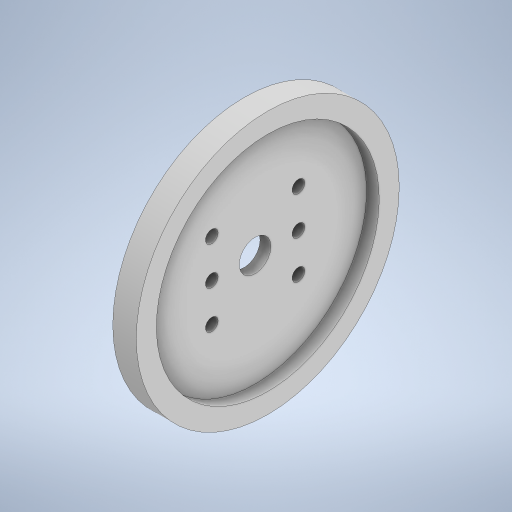
# Autodesk Inventor part: 4ax_plate_joint
Saved by Autodesk Inventor 2024 (Build 280153000, 153)
## iProperties
Created: 2025-12-19
Part Number: 4ax_plate_joint
Material: Generic
Document SubType Name: Modeling
Designer: schar
Density: 1 g/cm^3
Appearance: Default
Author: schar
Autodesk Inventor part; units mm, degrees
ref_plane "YZ Plane" through (0, 0, 0) normal (1, 0, 0) x (0, 1, 0)
ref_plane "XZ Plane" through (0, 0, 0) normal (0, 1, 0) x (-1, 0, 0)
ref_plane "XY Plane" through (0, 0, 0) normal (0, 0, 1) x (1, 0, 0)
sketch "Sketch1" plane through (0, 0, 0) normal (1, 0, 0) x (0, 1, 0)
  line L0 (0, 0) -> (0, -24.25)
  line L1 (0, 0) -> (0, 24.25)
  line L2 (0, 0) -> (33.993, 0)
  circle A0 centre (33.993, 0) radius 51.7565
  circle A1 centre (33.993, 0) radius 43.8815
  dimension "d0" = 24.25
  dimension "d1" = 24.25
  dimension "d2" = 33.993
  dimension "d3" = 103.513
  dimension "d17" = 87.763
  constraints: 6 end point, 2 centre point, 2 vertical, 1 coincident, 1 horizontal
  measures "d0" distance of L0.start L0.end
  measures "d1" distance of L0.start L1.end
  measures "d2" distance of L0.start L2.end
  measures "d3" diameter of A0
  measures "d17" diameter of A1
extrude "Extrusion1" add sketch "Sketch1" along normal blind 9.271
sketch "Sketch5" plane through (0, 33.993, 0) normal (-1, 0, 0) x (0, 0, 1)
  circle A0 centre (0, 0) radius 43.8815
  point P0 (0, -33.993)
  constraints: 1 centre point
extrude "Extrusion5" add sketch "Sketch5" against normal blind 4.271
sketch "Sketch6" plane through (4.271, 33.993, 0) normal (1, 0, 0) x (0, 0, -1)
  line L0 (0, 0) -> (17.056, 0)
  line L1 (0, 0) -> (-17.056, 0)
  circle A0 centre (-17.056, 0) radius 2.5
  circle A1 centre (17.056, 0) radius 2.5
  circle A2 centre (0, 0) radius 6.25
  line L2 (-17.056, 0) -> (-17.056, -15)
  line L3 (-17.056, 0) -> (-17.056, 15)
  line L4 (17.056, 0) -> (17.056, 15)
  line L5 (17.056, 0) -> (17.056, -15)
  circle A3 centre (-17.056, 15) radius 2.5
  circle A4 centre (-17.056, -15) radius 2.5
  circle A5 centre (17.056, 15) radius 2.5
  circle A6 centre (17.056, -15) radius 2.5
  point P0 (0, -33.993)
  dimension "d22" = 17.056
  dimension "d23" = 17.056
  dimension "d24" = 5
  dimension "d25" = 5
  dimension "d26" = 12.5
  dimension "d29" = 15
  dimension "d30" = 15
  dimension "d31" = 15
  dimension "d32" = 15
  dimension "d33" = 5
  dimension "d34" = 5
  dimension "d35" = 5
  dimension "d36" = 5
  constraints: 12 end point, 7 centre point, 7 coincident, 4 vertical, 2 horizontal
  measures "d22" distance of L0.start L0.end
  measures "d23" distance of L0.start L1.end
  measures "d24" diameter of A0
  measures "d25" diameter of A1
  measures "d26" diameter of A2
  measures "d29" distance of L2.start L2.end
  measures "d30" distance of L2.start L3.end
  measures "d31" distance of L4.start L4.end
  measures "d32" distance of L4.start L5.end
  measures "d33" diameter of A3
  measures "d34" diameter of A4
  measures "d35" diameter of A5
  measures "d36" diameter of A6
extrude "Extrusion6" cut sketch "Sketch6" against normal blind 4.271
body "Solid1"
